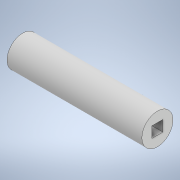
# Autodesk Inventor part: NeveRestVex
Saved by Autodesk Inventor 2020 (Build 240168000, 168)
## iProperties
Created: 2019-10-09
Part Number: NeveRestVex
Material: Generic
Document SubType Name: Modeling
Designer: robotics
Density: 1 g/cm^3
Appearance: Default
Author: robotics
Autodesk Inventor part; units mm, degrees
ref_plane "YZ Plane" through (0, 0, 0) normal (1, 0, 0) x (0, 1, 0)
ref_plane "XZ Plane" through (0, 0, 0) normal (0, 1, 0) x (-1, 0, 0)
ref_plane "XY Plane" through (0, 0, 0) normal (0, 0, 1) x (1, 0, 0)
sketch "Sketch1" plane through (0, 0, 0) normal (1, 0, 0) x (0, 1, 0)
  circle A0 centre (0, 0) radius 5.3975
  circle A1 centre (0, 0) radius 3.175
  line L0 (-3.175, 0) -> (2.413, 0) construction
  line L1 (2.413, 0) -> (2.413, -2.0635)
  line L2 (2.413, 0) -> (2.413, 2.0635)
  dimension "d0" = 10.795
  dimension "d1" = 6.35
  dimension "d2" = 5.588
  constraints: 6 end point, 3 point on circle, 2 centre point, 2 coincident, 1 horizontal, 1 point on line, 1 vertical
  measures "d0" diameter of A0
  measures "d1" diameter of A1
  measures "d2" distance of L0.start L0.end
extrude "Extrusion1" add sketch "Sketch1" along normal blind 25.4 contours A0 | A1 L1 L2 picked at (2.5514, -1.1687)
sketch "Sketch2" plane through (25.4, 0, 0) normal (1, 0, 0) x (0, 0, -1)
  circle A0 centre (0, 0) radius 5.3975
  dimension "d11" = 10.795
  constraints: 1 centre point, 1 coincident
  measures "d11" diameter of A0
extrude "Extrusion2" add sketch "Sketch2" along normal blind 2.54
sketch "Sketch3" plane through (27.94, 0, 0) normal (1, 0, 0) x (0, 0, -1)
  arc A0 (-2.0635, 2.413) -> (2.0635, 2.413) centre (0, 0) ccw projected
  circle A1 centre (0, 0) radius 5.3975
  line L0 (1.905, -1.905) -> (-1.905, -1.905)
  line L1 (-1.905, -1.905) -> (-1.905, 1.905)
  line L2 (-1.905, 1.905) -> (1.905, 1.905)
  line L3 (1.905, 1.905) -> (1.905, -1.905)
  line L4 (1.905, -1.905) -> (-1.905, 1.905) construction
  line L5 (-1.905, -1.905) -> (1.905, 1.905) construction
  dimension "d7" = 3.81
  dimension "d8" = 3.81
  dimension "d12" = 10.795
  constraints: 12 end point, 2 midpoint, 2 parallel, 1 centre point, 1 coincident, 1 horizontal, 1 perpendicular
  measures "d7" distance of L1.end L2.end
  measures "d8" distance of L2.end L0.start
  measures "d12" diameter of A1
extrude "Extrusion3" add sketch "Sketch3" along normal blind 19.05
body "Solid1"
